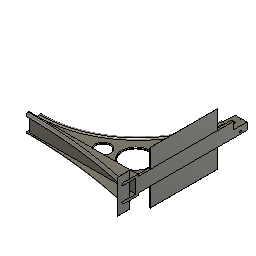
support_etagére_bureau (Autodesk Fusion 360 design; units mm, degrees)
Autodesk Fusion 360 part; units mm, degrees
sketch "Esquisse1" plane through (0, 0, 0) normal (1, 0, 0) x (0, 0, -1)
  line L0 (-92.2, 13.7) -> (92.2, 13.7)
  line L1 (92.2, 13.7) -> (92.2, -13.7)
  line L2 (92.2, -13.7) -> (-92.2, -13.7)
  line L3 (-92.2, -13.7) -> (-92.2, 13.7)
  line L4 (-92.2, 13.7) -> (92.2, -13.7) construction
  line L5 (92.2, 13.7) -> (-92.2, -13.7) construction
  line L6 (-112.6, 10.2) -> (-71.8, 10.2)
  line L7 (-71.8, 10.2) -> (-71.8, -10.2)
  line L8 (-71.8, -10.2) -> (-112.6, -10.2)
  line L9 (-112.6, -10.2) -> (-112.6, 10.2)
  line L10 (-112.6, 10.2) -> (-71.8, -10.2) construction
  line L11 (-71.8, 10.2) -> (-112.6, -10.2) construction
  point P0 (-92.2, 0)
  dimension "d5" = 184.4
  dimension "d6" = 27.4
  dimension "d7" = 40.8
  dimension "d8" = 20.4
  constraint horizontal L0
  constraint perpendicular L0 L1
  constraint parallel L0 L2
  constraint parallel L1 L3
  constraint coincident L4 origin
  constraint coincident L5 origin
  constraint horizontal L6
  constraint perpendicular L6 L7
  constraint parallel L6 L8
  constraint parallel L7 L9
  constraint coincident L10 P0
  constraint coincident L11 P0
  constraint midpoint L3 P0
  measures "d5" distance of L1.end L2.end
  measures "d7" distance of L7.end L8.end
  measures "d8" distance of L6.end L7.end
extrude "Extrusion1" add sketch "Esquisse1" along normal blind 160 contours L0 L1 L2 L3 L6 L7 L8
sketch "Esquisse2" plane through (0, 13.7, 0) normal (0, 1, 0) x (-1, 0, 0)
  line L0 (0, -92.2) -> (0, 92.2)
  line L1 (0, 92.2) -> (-160, 92.2)
  line L2 (-160, 92.2) -> (-160, -92.2)
  line L3 (-160, -92.2) -> (0, -92.2)
  circle A0 centre (1, -92.7) radius 147
  circle A1 centre (1, -92.7) radius 143.5
  circle A2 centre (-126, 37.8) radius 20
  line L4 (-145.9991, -92.2) -> (0, -92.2)
  line L5 (0, -92.2) -> (0, 1466.5539)
  line L6 (0, -92.2) -> (-156.5, -92.2)
  line L7 (-156.5, -92.2) -> (-156.5, 68.3)
  line L8 (-156.5, 68.3) -> (0, 68.3)
  line L9 (0, 68.3) -> (0, -92.2)
  line L10 (0, -92.2) -> (0, 92.2)
  circle A3 centre (-89, 49.05) radius 10.5
  circle A4 centre (-137.25, 0.8) radius 10.5
  circle A5 centre (0, 770.052) radius 696.502
  dimension "d11" = 294
  dimension "d12" = 184.9
  dimension "d13" = 161
  dimension "d20" = 40
  dimension "d45" = 160.5
  dimension "d46" = 156.5
  dimension "d109" = 21
  dimension "d110" = 21
  dimension "d111" = 37
  dimension "d112" = 19.25
  dimension "d123" = 19.25
  dimension "d124" = 37
  dimension "d133" = 34
  dimension "d136" = 677.852
  dimension "d137" = 1393.0039
  dimension "d138" = 30.5
  dimension "d140" = 160
  constraint horizontal L4
  constraint vertical L5
  constraint coincident L0 L5.end
  constraint coincident A0 L4.start
  constraint coincident L3 L4.start
  constraint horizontal L6
  constraint vertical L7
  constraint horizontal L8
  constraint vertical L9
  constraint coincident L5.end A5
  measures "d11" diameter of A0
  measures "d12" distance of L1 A0.centre
  measures "d13" distance of L2 A0.centre
  measures "d20" diameter of A2
  measures "d45" distance of L6 L8
  measures "d46" distance of L7 L10
  measures "d109" diameter of A3
  measures "d110" diameter of A4
  measures "d111" vertical distance of A2.centre A4.centre
  measures "d112" distance of L7 A4.centre
  measures "d123" distance of L8 A3.centre
  measures "d124" horizontal distance of A2.centre A3.centre
  measures "d133" distance of L2 A2.centre
  measures "d136" distance of L1 A5.centre
  measures "d137" diameter of A5
  measures "d138" distance of A2.centre L8
  measures "d140" distance of L2 A5.centre
extrude "Extrusion2" cut sketch "Esquisse2" against normal blind 27.4 contours L0 L3 A1 L4 L5 L6 L9 L10 | L0 L1 L2 L5 L10 A5 | A2 | A3 | A4 picked at (-6.7589, 2.6035)
sketch "Esquisse4" plane through (0, -13.7, 0) normal (0, -1, 0) x (1, 0, 0)
  arc A0 (142.4991, -92.2) -> (0, 50.7965) centre (-1, -92.7) ccw
  line L0 (142.4991, -92.2) -> (160, -92.2)
  line L1 (160, -92.2) -> (160, 92.1766)
  line L2 (0, 73.55) -> (0, 50.7965)
  line L3 (156.5, -92.2) -> (0, -92.2)
  line L4 (0, -92.2) -> (0, 68.3)
  line L5 (0, 68.3) -> (156.5, 68.3)
  line L6 (156.5, 68.3) -> (156.5, -92.2)
  line L7 (0, -92.2) -> (0, 1466.5539)
  line L8 (145.9991, -92.2) -> (0, -92.2)
  circle A1 centre (-1, -92.7) radius 143.5
  circle A2 centre (-1, -92.7) radius 147
  circle A3 centre (126, 37.8) radius 20
  circle A4 centre (137.25, 0.8) radius 10.5
  circle A5 centre (89, 49.05) radius 10.5
  arc A6 (0, 73.55) -> (160, 92.1766) centre (0, 770.052) ccw
  dimension "d43" = 156.5
  dimension "d44" = 160.5
  dimension "d51" = 3.5
  dimension "d52" = 294
  constraint horizontal L3
  constraint vertical L4
  constraint horizontal L5
  constraint vertical L6
  constraint coincident L2 L4.end
  constraint coincident L0 L3.start
  constraint concentric A0 A1
  measures "d43" distance of L6 L7
  measures "d44" distance of L5 L8
  measures "d52" diameter of A2
extrude "Extrusion7" cut sketch "Esquisse4" against normal blind 12.45 contours L0 L2 L3 L4 L5 L6 L7 A2 | A3 | A4 | A5
extrude "Extrusion9" cut sketch "Esquisse2" against normal blind 12.45 contours L0 L3 A0 L5 L6 L7 L8 L9 L10 | A2 | A3 | A4
extrude "Extrusion10" cut sketch "Esquisse4" against normal blind 10.7 contours A0 L0 L2 L3 L4 L7 L8 A1 A2 | L0 L2 L3 L4 L7 L8 A1 A2
extrude "Extrusion11" cut sketch "Esquisse2" against normal blind 10.7 contours L0 L3 A0 A1 L4 L5 L6 L9 L10 | L0 L3 A0 A1 L4 L5 L6 L9 L10
sketch "Esquisse3" plane through (160, 0, 0) normal (1, 0, 0) x (0, 0, -1)
  line L0 (-71.8, 10.2) -> (-71.8, -10.2)
  line L1 (-71.8, -10.2) -> (-92.1766, -10.2)
  line L2 (-92.1766, -13.7) -> (92.2, -13.7)
  line L3 (92.2, -13.7) -> (92.2, 13.7)
  circle A0 centre (82.2, 0) radius 1.25
  line L4 (-92.1766, 10.2) -> (-71.8, 10.2)
  line L5 (92.2, 13.7) -> (-92.1766, 13.7)
  circle A1 centre (82.2, 0) radius 3.125
  line L6 (49.1, -1) -> (49.1, 1)
  line L7 (-50.7865, 38.6391) -> (49.2135, 38.6391)
  line L8 (49.2135, 38.6391) -> (49.2135, -38.6391)
  line L9 (49.2135, -38.6391) -> (-50.7865, -38.6391)
  line L10 (-50.7865, -38.6391) -> (-50.7865, 38.6391)
  line L11 (-50.7865, 38.6391) -> (49.2135, -38.6391) construction
  line L12 (49.2135, 38.6391) -> (-50.7865, -38.6391) construction
  circle A2 centre (82.2, 7) radius 1.25
  circle A3 centre (82.2, 7) radius 3.125
  circle A4 centre (82.2, -7) radius 3.125
  circle A5 centre (82.2, -7) radius 1.25
  line L13 (92.2, -0.1) -> (72.2, -0.1)
  line L14 (72.2, -0.1) -> (72.2, 13.7)
  line L15 (72.2, 13.7) -> (92.2, 13.7)
  line L16 (92.2, 13.7) -> (92.2, -0.1)
  line L17 (-81.2407, -24.7806) -> (-98.7593, -24.7806)
  line L18 (-98.7593, -24.7806) -> (-98.7593, 24.7806)
  line L19 (-98.7593, 24.7806) -> (-81.2407, 24.7806)
  line L20 (-81.2407, 24.7806) -> (-81.2407, -24.7806)
  line L21 (-81.2407, -24.7806) -> (-98.7593, 24.7806) construction
  line L22 (-98.7593, -24.7806) -> (-81.2407, 24.7806) construction
  line L23 (92.2, 13.7) -> (-68.3, 13.7)
  line L24 (-68.3, 13.7) -> (-68.3, 10.7)
  line L25 (-68.3, 10.7) -> (92.2, 10.7)
  line L26 (92.2, 10.7) -> (92.2, 13.7)
  line L27 (92.2, -13.7) -> (-68.3, -13.7)
  line L28 (-68.3, -13.7) -> (-68.3, -10.7)
  line L29 (-68.3, -10.7) -> (92.2, -10.7)
  line L30 (92.2, -10.7) -> (92.2, -13.7)
  line L31 (-92.1766, -10.2) -> (-92.1766, -13.7)
  line L32 (-92.1766, 13.7) -> (-92.1766, 10.2)
  point P0 (-0.7865, 0)
  point P1 (-90, 0)
  dimension "d27" = 2.5
  dimension "d28" = 10
  dimension "d29" = 13.7
  dimension "d69" = 6.25
  dimension "d86" = 100
  dimension "d101" = 2.5
  dimension "d102" = 6.25
  dimension "d103" = 2.5
  dimension "d104" = 6.25
  dimension "d105" = 7
  dimension "d106" = 7
  dimension "d113" = 20
  dimension "d114" = 13.8
  dimension "d115" = 13.6
  dimension "d142" = 3
  dimension "d143" = 160.5
  dimension "d144" = 160.5
  dimension "d145" = 3
  constraint concentric A0 A1
  constraint horizontal L7
  constraint perpendicular L7 L8
  constraint parallel L7 L9
  constraint parallel L8 L10
  constraint coincident L11 P0
  constraint coincident L12 P0
  constraint concentric A2 A3
  constraint concentric A4 A5
  constraint horizontal L13
  constraint vertical L14
  constraint horizontal L15
  constraint vertical L16
  constraint horizontal L17
  constraint perpendicular L17 L18
  constraint parallel L17 L19
  constraint parallel L18 L20
  constraint coincident L21 P1
  constraint coincident L22 P1
  constraint horizontal L23
  constraint vertical L24
  constraint horizontal L25
  constraint vertical L26
  constraint coincident L3.end L5.start
  constraint horizontal L27
  constraint vertical L28
  constraint horizontal L29
  constraint vertical L30
  constraint coincident L2.end L3.start
  measures "d27" diameter of A0
  measures "d28" distance of L3 A0.centre
  measures "d29" distance of L2 A0.centre
  measures "d69" diameter of A1
  measures "d86" distance of L8 L10
  measures "d101" diameter of A2
  measures "d102" diameter of A3
  measures "d103" diameter of A5
  measures "d104" diameter of A4
  measures "d105" distance of A0.centre A4.centre
  measures "d106" distance of A0.centre A2.centre
  measures "d113" distance of L14 L16
  measures "d114" distance of L13 L15
  measures "d115" distance of L2 L13
  measures "d142" distance of L3.end L25.end
  measures "d143" distance of L24 L26
  measures "d144" distance of L2.end L27.end
  measures "d145" distance of L2.end L29.end
extrude "Extrusion12" cut sketch "Esquisse3" against normal blind 160 contours A2 | A5
fillet "Congé4" radius 1.75 4 edges at (100.6464, -3, 8.5929) (100.6464, 3, 8.5929) (103.1213, -3, 11.0678) (103.1213, 3, 11.0678)
fillet "Congé5" radius 5.25 2 edges at (156.5, 1.25, -11.95) (156.5, -1.25, -11.95)
sketch "Esquisse9" plane through (156.5, 0, 0) normal (-1, 0, 0) x (0, 0, 1)
  line L0 (68.3, -6.5) -> (-81.0544, -6.5)
  arc A0 (-83.3456, -6.5) -> (-81.0544, -6.5) centre (-82.2, -7) ccw
  line L1 (-83.3456, -6.5) -> (-92.2, -6.5)
  line L2 (-92.2, -6.5) -> (-92.2, -13.7)
  line L3 (-92.2, -13.7) -> (68.3, -13.7)
  line L4 (68.3, -13.7) -> (68.3, -6.5)
  circle A1 centre (-82.2, -7) radius 3.125
  circle A2 centre (-82.2, 7) radius 3.125
  dimension "d146" = 6.25
  dimension "d147" = 6.25
  constraint concentric A0 A1
  measures "d146" diameter of A1
  measures "d147" diameter of A2
extrude "Extrusion23" cut sketch "Esquisse9" along normal blind 3.5 contours L0 A0 L1 A1 | L0 A0 L1 A1 | A2
chamfer "Chanfrein7" distance 1.5 angle 45 2 edges at (156.5, 6.548, -81.0346) (156.5, -7.452, -81.0346)
extrude "Extrusion24" cut sketch "Esquisse3" against normal blind 3.5 contours L5 L10 L23 L24 L25 | L2 L10 L27 L28 L29 | L5 L8 L10 L23 L25 | L2 L8 L10 L27 L29 | L5 L8 L14 L23 L25 | L2 L3 L8 L27 L29 L30 | L3 L5 L14 L15 L16 L23 L25 L26
fillet "Congé8" radius 7 6 edges at (156.5, 8.6, 68.3) (154.9623, 2.7877, 68.3) (75.625, 1.25, 68.3) (156.5, -8.6, 68.3) (154.9623, -2.7877, 68.3) (75.625, -1.25, 68.3)
fillet "Congé10" radius 3.5 2 edges at (80.5403, -13.7, 78.2223) (80.5403, 13.7, 78.2223)
fillet "Congé6" radius 0.5 8 edges at (80, 13.7, 68.3) (80, -13.7, 68.3) (154.4497, 10.7, 66.2497) (156.5, 10.7, -15.45) (156.5, -10.7, -15.45) (154.4497, -10.7, 66.2497) (154.75, -10.7, 68.3) (154.75, 10.7, 68.3)
fillet "Congé13" radius 1 6 edges at (144.6465, 1.25, 30.5677) (98.7894, 1.25, 45.253) (98.7894, -1.25, 52.847) (144.6465, -1.25, 45.0323) (147.0394, -1.25, 4.597) (147.0394, 1.25, -2.997)
extrude "Extrusion17" add sketch "Esquisse3" against normal blind 0.2 contours L1 L2 L4 L5 L17 L18 L19 L20 L31 L32 | L4 L5 L20 L32 | L1 L2 L20 L31 | L5 L7 L8 L10 L23 | L5 L8 L10 L23 L25 | L2 L8 L10 L27 L29 | L2 L8 L9 L10 L27 | L8 L10 L25 L29
fillet "Congé9" radius 3.5 2 edges at (103.1213, 1.25, 11.0678) (103.1213, -1.25, 11.0678)
extrude "Extrusion20" cut sketch "Esquisse3" against normal blind 50 contours L3 L5 L14 L15 L16 L23 L25 L26 | L3 A1 L13 L14 L16 L25 | A0 A1 L13 | A0 L13 | A2 | A3 picked at (79.708, 0.111) picked at (82.1239, 0.365)
chamfer "Chanfrein6" distance 3 angle 45 1 edges at (0, 0, 71.8)
sketch "Esquisse7" plane through (0, -0.1, 0) normal (0, 1, 0) x (-1, 0, 0)
  arc A0 (-141.0282, -72.2) -> (-142.4991, -92.2) centre (1, -92.7) ccw
  line L0 (-141.0282, -72.2) -> (-160, -72.2)
  line L1 (-160, -72.2) -> (-160, -92.2)
  line L2 (-160, -92.2) -> (-142.4991, -92.2)
  circle A1 centre (-151, -82.2) radius 1.5
  line L3 (-156.5, -92.2) -> (0, -92.2)
  line L4 (-160, -92.2) -> (-160, 68.3)
  dimension "d122" = 3
  dimension "d132" = 10
  dimension "d155" = 9
  measures "d122" diameter of A1
  measures "d132" distance of A1.centre L3
  measures "d155" distance of A1.centre L4
extrude "Extrusion21" cut sketch "Esquisse7" against normal blind 20 contours A1
sketch "Esquisse8" plane through (0, -1.25, 0) normal (0, -1, 0) x (1, 0, 0)
  line L0 (148.1623, -92.2) -> (151.25, -92.2)
  line L1 (151.25, -80.721) -> (151.25, 61.3)
  circle A0 centre (151, -82.2) radius 4
  arc A1 (148.1623, -92.2) -> (0, 56.4598) centre (-1, -92.7) ccw
  line L2 (151.25, 61.3) -> (0, 61.3)
  line L3 (0, 61.3) -> (0, 56.4598)
  circle A2 centre (137.25, 0.8) radius 11.5
  circle A3 centre (89, 49.05) radius 11.5
  circle A4 centre (126, 37.8) radius 21
  arc A5 (151.25, -80.721) -> (151.25, -83.679) centre (151, -82.2) ccw
  line L4 (160, -92.2) -> (160, 68.3)
  line L5 (151.25, -92.2) -> (151.25, -83.679)
  dimension "d130" = 8
  dimension "d131" = 10
  dimension "d156" = 9
  measures "d130" diameter of A0
  measures "d131" distance of L0 A0.centre
  measures "d156" distance of A0.centre L4
extrude "Extrusion22" cut sketch "Esquisse8" along normal blind 10 contours L1 A0 A1 A5 L5 | A0 A1 | L1 A0 A5 L5
equation "largeur_hors_tout = 308 mm" comment "doit etre 308"
equation "epaisseur_montant = 20.4 mm"
equation "hauteur_support = 160 mm"
equation "epaisseur_min = 3.5 mm"
equation "d5 = largeur_hors_tout / 2 + epaisseur_montant + chevauchement / 2"
equation "d6 = epaisseur_min * 2 + epaisseur_montant"
equation "d7 = epaisseur_montant * 2"
equation "d8 = epaisseur_montant"
equation "d9 = hauteur_support"
equation "d11 = largeur_hors_tout - 4 * epaisseur_min"
equation "d12 = largeur_hors_tout / 2 + epaisseur_montant + epaisseur_min * 2 + hauteur_nervure"
equation "d13 = d11 / 2 + epaisseur_min * 2 + hauteur_nervure * 2"
equation "d14 = -hauteur_nervure"
equation "hauteur_nervure = epaisseur_min"
equation "d16 = -d6"
equation "d21 = d20 / 2 + epaisseur_min * 4 + epaisseur_montant"
equation "diametre_vis = 2.5 mm"
equation "d27 = diametre_vis"
equation "d28 = d113 / 2"
equation "d29 = d6 / 2"
equation "diametre_lamage_vis = 2.5 * diametre_vis"
equation "d41 = -( epaisseur_montant / 2 + epaisseur_min / 2 ) - 0.5 mm"
equation "d43 = d46"
equation "d44 = d45"
equation "d45 = ( largeur_hors_tout + chevauchement ) / 2 - epaisseur_min"
equation "d46 = hauteur_support - epaisseur_min"
equation "d49 = d41"
equation "d51 = -d14"
equation "d52 = d11"
equation "d53 = d41 + epaisseur_min / 2"
equation "d55 = d53"
equation "d59 = epaisseur_min / 2"
equation "d60 = -hauteur_support"
equation "d64 = epaisseur_min * 1.5"
equation "d69 = d102"
equation "d75 = 4 mm"
equation "d78 = d75 / 2 + epaisseur_min / 2"
equation "d90 = epaisseur_min * 2"
equation "d92 = epaisseur_min"
equation "d98 = epaisseur_min"
equation "d101 = diametre_vis"
equation "d102 = diametre_lamage_vis"
equation "d103 = diametre_vis"
equation "d104 = d102"
equation "d106 = d105"
equation "d112 = d123"
equation "d114 = d6 / 2 + 0.1 mm"
equation "d115 = d6 / 2 - 0.1 mm"
equation "chevauchement = 20 mm" comment "doit etre 20"
equation "d123 = d109 / 2 + epaisseur_min * 2.5"
equation "d131 = d132"
equation "d132 = d113 / 2"
equation "d133 = d21 - epaisseur_montant"
equation "d136 = d137 / 2 - epaisseur_montant + epaisseur_min / 2"
equation "d137 = 2 * ( ( ( hauteur_support - epaisseur_montant * 2 ) ^ 2 ) / epaisseur_montant )"
equation "d138 = d20 / 2 + epaisseur_min * 3"
equation "d140 = hauteur_support"
equation "d142 = epaisseur_min - 0.5 mm"
equation "d143 = d45"
equation "d144 = d143"
equation "d145 = d142"
equation "d146 = d102"
equation "d147 = d102"
equation "d148 = epaisseur_min"
equation "d151 = -epaisseur_min"
equation "d156 = d155"
